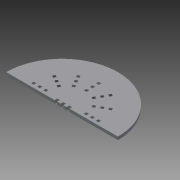
# Autodesk Inventor part: base
Saved by Autodesk Inventor 2014 SP1 (Build 180222100, 222)
## iProperties
Created: 2015-02-17
Part Number: base
Material: Generic
Document SubType Name: Modeling
Designer: Erin
Density: 1 g/cm^3
Appearance: Default
Author: Erin
Autodesk Inventor part; units mm, degrees
ref_plane "YZ Plane" through (0, 0, 0) normal (1, 0, 0) x (0, 1, 0)
ref_plane "XZ Plane" through (0, 0, 0) normal (0, 1, 0) x (-1, 0, 0)
ref_plane "XY Plane" through (0, 0, 0) normal (0, 0, 1) x (1, 0, 0)
sketch "slots" plane through (0, 0, 0) normal (0, 0, 1) x (1, 0, 0)
  line L0 (61.2067, 31.1571) -> (64.2567, 31.1571)
  line L1 (64.2567, 31.1571) -> (64.2567, 28.1071)
  line L2 (64.2567, 28.1071) -> (61.2067, 28.1071)
  line L3 (61.2067, 28.1071) -> (61.2067, 31.1571)
  line L4 (68.9317, 33.8834) -> (68.9317, 26.9198) construction
  line L5 (67.4067, 31.1571) -> (70.4567, 31.1571)
  line L6 (70.4567, 31.1571) -> (70.4567, 28.1071)
  line L7 (70.4567, 28.1071) -> (67.4067, 28.1071)
  line L8 (67.4067, 28.1071) -> (67.4067, 31.1571)
  line L9 (73.6067, 31.1571) -> (76.6567, 31.1571)
  line L10 (76.6567, 31.1571) -> (76.6567, 28.1071)
  line L11 (76.6567, 28.1071) -> (73.6067, 28.1071)
  line L12 (73.6067, 28.1071) -> (73.6067, 31.1571)
  line L13 (68.9317, 28.1071) -> (68.9317, 27.1937) construction
  line L14 (77.0148, 29.5071) -> (60.408, 29.5071) construction
  point P0 (68.8645, 30.3856)
  dimension "d2" = 3.05
  dimension "d3" = 3.05
  dimension "d4" = 3.15
  dimension "d5" = 3.15
  measures "d2" distance of L1.end L2.end
  measures "d3" distance of L0.end L1.end
  measures "d4" distance between parallel lines of L8 L1
  measures "d5" distance between parallel lines of L12 L6
sketch "Sketch1" plane through (0, 0, 0) normal (0, 0, 1) x (1, 0, 0)
  line L0 (0, 40.2669) -> (0, -8.968) construction
  line L1 (-55, 0) -> (61.3149, 0) construction
  line L2 (0, 55) -> (22.0392, 55) construction
  arc A0 (55, 0) -> (-55, 0) centre (0, 0) ccw
  line L3 (-55, 0) -> (55, 0)
  line L4 (-8.8642, 4) -> (11.5268, 4) construction
  line L5 (-1.65, 22.275) -> (-1.65, 25.325)
  line L6 (-1.65, 25.325) -> (1.4, 25.325)
  line L7 (1.4, 25.325) -> (1.4, 22.275)
  line L8 (1.4, 22.275) -> (-1.65, 22.275)
  line L9 (-4.3763, 30) -> (2.5873, 30) construction
  line L10 (-1.65, 28.475) -> (-1.65, 31.525)
  line L11 (-1.65, 31.525) -> (1.4, 31.525)
  line L12 (1.4, 31.525) -> (1.4, 28.475)
  line L13 (1.4, 28.475) -> (-1.65, 28.475)
  line L14 (-1.65, 34.675) -> (-1.65, 37.725)
  line L15 (-1.65, 37.725) -> (1.4, 37.725)
  line L16 (1.4, 37.725) -> (1.4, 34.675)
  line L17 (1.4, 34.675) -> (-1.65, 34.675)
  line L18 (1.4, 30) -> (2.3134, 30) construction
  line L19 (0, 38.0831) -> (0, 21.4763) construction
  line L20 (7.7086, 20.6516) -> (9.2336, 23.293)
  line L21 (9.2336, 23.293) -> (11.8749, 21.768)
  line L22 (11.8749, 21.768) -> (10.3499, 19.1266)
  line L23 (10.3499, 19.1266) -> (7.7086, 20.6516)
  line L24 (9.21, 28.7048) -> (15.2406, 25.223) construction
  line L25 (10.8086, 26.021) -> (12.3336, 28.6623)
  line L26 (12.3336, 28.6623) -> (14.9749, 27.1373)
  line L27 (14.9749, 27.1373) -> (13.4499, 24.496)
  line L28 (13.4499, 24.496) -> (10.8086, 26.021)
  line L29 (13.9086, 31.3903) -> (15.4336, 34.0317)
  line L30 (15.4336, 34.0317) -> (18.0749, 32.5067)
  line L31 (18.0749, 32.5067) -> (16.5499, 29.8653)
  line L32 (16.5499, 29.8653) -> (13.9086, 31.3903)
  line L33 (14.2124, 25.8167) -> (15.0034, 25.36) construction
  line L34 (17.0416, 33.5169) -> (8.7382, 19.1349) construction
  line L35 (15.0016, 14.5664) -> (17.643, 16.0914)
  line L36 (17.643, 16.0914) -> (19.168, 13.4501)
  line L37 (19.168, 13.4501) -> (16.5266, 11.9251)
  line L38 (16.5266, 11.9251) -> (15.0016, 14.5664)
  line L39 (20.3285, 20.79) -> (23.8103, 14.7594) construction
  line L40 (20.371, 17.6664) -> (23.0123, 19.1914)
  line L41 (23.0123, 19.1914) -> (24.5373, 16.5501)
  line L42 (24.5373, 16.5501) -> (21.896, 15.0251)
  line L43 (21.896, 15.0251) -> (20.371, 17.6664)
  line L44 (25.7403, 20.7664) -> (28.3817, 22.2914)
  line L45 (28.3817, 22.2914) -> (29.9067, 19.6501)
  line L46 (29.9067, 19.6501) -> (27.2653, 18.1251)
  line L47 (27.2653, 18.1251) -> (25.7403, 20.7664)
  line L48 (23.2167, 15.7876) -> (23.6733, 14.9966) construction
  line L49 (29.5169, 21.0416) -> (15.1349, 12.7382) construction
  line L50 (18.275, 5.65) -> (21.325, 5.65)
  line L51 (21.325, 5.65) -> (21.325, 2.6)
  line L52 (21.325, 2.6) -> (18.275, 2.6)
  line L53 (18.275, 2.6) -> (18.275, 5.65)
  line L54 (26, 8.3763) -> (26, 1.4127) construction
  line L55 (24.475, 5.65) -> (27.525, 5.65)
  line L56 (27.525, 5.65) -> (27.525, 2.6)
  line L57 (27.525, 2.6) -> (24.475, 2.6)
  line L58 (24.475, 2.6) -> (24.475, 5.65)
  line L59 (30.675, 5.65) -> (33.725, 5.65)
  line L60 (33.725, 5.65) -> (33.725, 2.6)
  line L61 (33.725, 2.6) -> (30.675, 2.6)
  line L62 (30.675, 2.6) -> (30.675, 5.65)
  line L63 (26, 2.6) -> (26, 1.6866) construction
  line L64 (34.0831, 4) -> (17.4763, 4) construction
  line L65 (-10.5664, 19.0016) -> (-12.0914, 21.643)
  line L66 (-12.0914, 21.643) -> (-9.4501, 23.168)
  line L67 (-9.4501, 23.168) -> (-7.9251, 20.5266)
  line L68 (-7.9251, 20.5266) -> (-10.5664, 19.0016)
  line L69 (-16.79, 24.3285) -> (-10.7594, 27.8103) construction
  line L70 (-13.6664, 24.371) -> (-15.1914, 27.0123)
  line L71 (-15.1914, 27.0123) -> (-12.5501, 28.5373)
  line L72 (-12.5501, 28.5373) -> (-11.0251, 25.896)
  line L73 (-11.0251, 25.896) -> (-13.6664, 24.371)
  line L74 (-16.7664, 29.7403) -> (-18.2914, 32.3817)
  line L75 (-18.2914, 32.3817) -> (-15.6501, 33.9067)
  line L76 (-15.6501, 33.9067) -> (-14.1251, 31.2653)
  line L77 (-14.1251, 31.2653) -> (-16.7664, 29.7403)
  line L78 (-11.7876, 27.2167) -> (-10.9966, 27.6733) construction
  line L79 (-17.0416, 33.5169) -> (-8.7382, 19.1349) construction
  line L80 (-16.6516, 11.7086) -> (-19.293, 13.2336)
  line L81 (-19.293, 13.2336) -> (-17.768, 15.8749)
  line L82 (-17.768, 15.8749) -> (-15.1266, 14.3499)
  line L83 (-15.1266, 14.3499) -> (-16.6516, 11.7086)
  line L84 (-24.7048, 13.21) -> (-21.223, 19.2406) construction
  line L85 (-22.021, 14.8086) -> (-24.6623, 16.3336)
  line L86 (-24.6623, 16.3336) -> (-23.1373, 18.9749)
  line L87 (-23.1373, 18.9749) -> (-20.496, 17.4499)
  line L88 (-20.496, 17.4499) -> (-22.021, 14.8086)
  line L89 (-27.3903, 17.9086) -> (-30.0317, 19.4336)
  line L90 (-30.0317, 19.4336) -> (-28.5067, 22.0749)
  line L91 (-28.5067, 22.0749) -> (-25.8653, 20.5499)
  line L92 (-25.8653, 20.5499) -> (-27.3903, 17.9086)
  line L93 (-21.8167, 18.2124) -> (-21.36, 19.0034) construction
  line L94 (-29.5169, 21.0416) -> (-15.1349, 12.7382) construction
  line L95 (-18.275, 2.35) -> (-21.325, 2.35)
  line L96 (-21.325, 2.35) -> (-21.325, 5.4)
  line L97 (-21.325, 5.4) -> (-18.275, 5.4)
  line L98 (-18.275, 5.4) -> (-18.275, 2.35)
  line L99 (-26, -0.3763) -> (-26, 6.5873) construction
  line L100 (-24.475, 2.35) -> (-27.525, 2.35)
  line L101 (-27.525, 2.35) -> (-27.525, 5.4)
  line L102 (-27.525, 5.4) -> (-24.475, 5.4)
  line L103 (-24.475, 5.4) -> (-24.475, 2.35)
  line L104 (-30.675, 2.35) -> (-33.725, 2.35)
  line L105 (-33.725, 2.35) -> (-33.725, 5.4)
  line L106 (-33.725, 5.4) -> (-30.675, 5.4)
  line L107 (-30.675, 5.4) -> (-30.675, 2.35)
  line L108 (-26, 5.4) -> (-26, 6.3134) construction
  line L109 (-34.0831, 4) -> (-17.4763, 4) construction
  line L110 (7.725, 0) -> (4.675, 0)
  line L111 (4.675, 0) -> (4.675, 3.05)
  line L112 (4.675, 3.05) -> (7.725, 3.05)
  line L113 (7.725, 3.05) -> (7.725, 0)
  line L114 (0, -2.7263) -> (0, 4.2373) construction
  line L115 (1.525, 0) -> (-1.525, 0)
  line L116 (-1.525, 0) -> (-1.525, 3.05)
  line L117 (-1.525, 3.05) -> (1.525, 3.05)
  line L118 (1.525, 3.05) -> (1.525, 0)
  line L119 (-4.675, 0) -> (-7.725, 0)
  line L120 (-7.725, 0) -> (-7.725, 3.05)
  line L121 (-7.725, 3.05) -> (-4.675, 3.05)
  line L122 (-4.675, 3.05) -> (-4.675, 0)
  line L123 (0, 3.05) -> (0, 3.9634) construction
  line L124 (-8.0831, 1.65) -> (8.5237, 1.65) construction
  point P0 (25, 0)
  point P1 (0, 4)
  dimension "d8" = 30
  dimension "d9" = 25
  dimension "d22" = 4
  dimension "d29" = 90
  dimension "d33" = 90
  constraints: 10 end point, 3 horizontal, 3 point on circle, 3 point on line, 3 vertical, 1 centre point, 1 coincident, 1 parallel, 1 perpendicular, 1 tangent, 8 other
  measures "d22" distance between parallel lines of L1 L4
extrude "Extrusion1" add sketch "Sketch1" along normal blind 3.1 contours L3 L113 L112 L111 L118 L117 L116 L122 L121 L120 A0
equation "\"d2\" = mat - kerf"
equation "\"d3\" = mat - kerf"
equation "\"d4\" = mat + kerf"
equation "\"d5\" = mat + kerf"
equation "\"d39\" = mat"
equation "\"mat\" = 3.1"
equation "\"kerf\" = 0.05"
body "Solid1"
